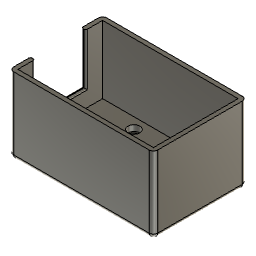
GPS Holder v3 (Autodesk Fusion 360 design; units mm, degrees)
Autodesk Fusion 360 part; units mm, degrees
sketch "Sketch1" plane through (0, 0, 0) normal (0, 0, 1) x (1, 0, 0)
  line L0 (0, 0) -> (160, 0)
  line L1 (160, 0) -> (160, 100)
  line L2 (160, 100) -> (0, 100)
  line L3 (0, 100) -> (0, 0)
  line L4 (-5, -5) -> (165, -5)
  line L5 (165, -5) -> (165, 105)
  line L6 (165, 105) -> (-5, 105)
  line L7 (-5, 105) -> (-5, -5)
  circle A0 centre (50, 87) radius 5
  circle A1 centre (50, 87) radius 7
  circle A2 centre (110, 87) radius 5
  circle A3 centre (110, 87) radius 7
  dimension "d1" = 160
  dimension "d2" = 100
  dimension "d3" = 14
  dimension "d4" = 10
  dimension "d5" = 14
  constraint horizontal L0
  constraint vertical L1
  constraint horizontal L2
  constraint vertical L3
  constraint coincident L0.start L3.end
  constraint horizontal L4
  constraint vertical L5
  constraint horizontal L6
  constraint vertical L7
  constraint concentric A0 A1
  constraint concentric A2 A3
  measures "d1" distance of L0.start L0.end
  measures "d2" distance of L0.start L2.end
  measures "d3" diameter of A1
  measures "d4" diameter of A2
  measures "d5" diameter of A3
extrude "Extrude1" add sketch "Sketch1" along normal blind 3 contours A1 makes body 1
extrude "Extrude2" add sketch "Sketch1" along normal blind 3 separate body contours A3 makes body 2
extrude "Extrude3" add sketch "Sketch1" along normal blind 10 contours L0 L1 L2 L3 bodies 1 2
extrude "Extrude4" add sketch "Sketch1" along normal blind 90 contours L4 L5 L6 L7 bodies 1
sketch "Sketch2" plane through (0, 0, 90) normal (0, 0, 1) x (-1, 0, 0)
  line L0 (0, 0) -> (0, -100)
  line L1 (0, -100) -> (-160, -100)
  line L2 (-160, -100) -> (-160, 0)
  line L3 (-160, 0) -> (0, 0)
  line L4 (5, -105) -> (5, 5)
  line L5 (5, 5) -> (-165, 5)
  line L6 (-165, 5) -> (-165, -105)
  line L7 (-165, -105) -> (5, -105)
  line L8 (5, -80) -> (0, -80)
  line L9 (0, -80) -> (0, -20)
  line L10 (0, -20) -> (5, -20)
  line L11 (5, -20) -> (5, -80)
  constraint horizontal L8
  constraint vertical L9
  constraint horizontal L10
  constraint vertical L11
  constraint coincident L0 L9.end
  constraint coincident L4 L8.start
extrude "Extrude5" cut sketch "Sketch2" against normal blind 60 contours L0 L4 L8 L9 L10 L11 bodies 1
fillet "Fillet1" radius 5 8 edges at (-5, -5, 45) (-5, 50, 0) (80, -5, 0) (165, -5, 45) (165, 50, 0) (165, 105, 45) (80, 105, 0) (-5, 105, 45) on bodies 1
fillet "Fillet1" radius 2 6 edges at (-5, 80, 60) (0, 80, 60) (-5, 20, 60) (0, 20, 60) (-5, 50, 30) (0, 50, 30) on bodies 1
